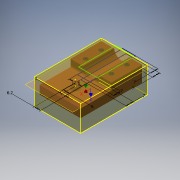
# Autodesk Inventor part: 17-0028-0109
Saved by Autodesk Inventor 2016 SP2 (Build 200236200, 236)
## iProperties
Created: 2017-12-29
Part Number: 17-0028-0109
Material: Copper
Document SubType Name: Modeling
Designer: Daan Giesen
Density: 8.94 g/cm^3
Appearance: Copper - Satin
Project: Digital PID Loop
Cost Center: 17-0028
User Status: CNC
Authority: Reichsöllner, Lukas
Mass: 216.263 g
Surface Area: 82.0629 cm^2
Volume: 24.1905 cm^3
Category: IOP
Company: Universiteit van Amsterdam
Author: Daan Giesen
Title: Digital PID Loop
Revision Number: A.1
Autodesk Inventor part; units mm, degrees
ref_plane "YZ Plane" through (0, 0, 0) normal (1, 0, 0) x (0, 1, 0)
ref_plane "XZ Plane" through (0, 0, 0) normal (0, 1, 0) x (-1, 0, 0)
sketch "Sketch1" plane through (0, 0, 0) normal (0, 0, 1) x (1, 0, 0)
  line L0 (0, 57) -> (0, -27) construction
  line L1 (-28, 0) -> (28, 0) construction
  line L2 (-20, 45) -> (20, 45)
  line L3 (20, 45) -> (20, -15)
  line L4 (20, -15) -> (-20, -15)
  line L5 (-20, -15) -> (-20, 45)
  line L6 (-20, 45) -> (20, -15) construction
  line L7 (20, 45) -> (-20, -15) construction
  point P0 (0, 0)
  point P1 (0, 15)
  dimension "d0" = 60
  dimension "d1" = 40
  dimension "d2" = 15
  constraints: 12 end point, 3 midpoint, 2 parallel, 1 horizontal, 1 perpendicular
  measures "d0" distance of L4.end L2.start
  measures "d1" distance of L3.end L4.end
  measures "d2" distance from line of L4 point (0, 0)
extrude "Extrusion1" add sketch "Sketch1" along normal blind 8
sketch "Sketch2" plane through (0, 0, 8) normal (0, 0, 1) x (1, 0, 0)
  point P0 (0, 0)
  point P1 (0, 0)
  constraints: 1 coincident
hole "Hole1" at (0, 0, 8) direction (0, 0, -1) diameter 8 end through all
sketch "Sketch3" plane through (0, 0, 8) normal (0, 0, 1) x (1, 0, 0)
  line L0 (-20, 15) -> (20, 15)
  line L1 (20, 15) -> (20, 45)
  line L2 (20, 45) -> (-20, 45)
  line L3 (-20, 45) -> (-20, 15)
  line L4 (-20, 15) -> (20, 45) construction
  line L5 (20, 15) -> (-20, 45) construction
  circle A0 centre (0, 0) radius 4 projected
  line L6 (20, 45) -> (-20, 45) projected
  line L7 (-20, 45) -> (-20, -15) projected
  line L8 (-20, -15) -> (20, -15) projected
  line L9 (20, -15) -> (20, 45) projected
  point P0 (0, 30)
  dimension "d12" = 30
  constraints: 12 end point, 2 midpoint, 2 parallel, 1 horizontal, 1 perpendicular
  measures "d12" distance between parallel lines of L2 L0
extrude "Extrusion2" add sketch "Sketch3" along normal blind 7 contours L3 L2 L1 L0
sketch "Sketch4" plane through (-20, 45, 0) normal (0, 1, 0) x (1, 0, 0)
  circle A0 centre (20, -16) radius 7.5
  line L0 (40, -15) -> (0, -15) projected
  line L1 (0, 0) -> (40, 0) projected
  point P0 (20, 0)
  point P1 (20, 0)
  dimension "d15" = 1
  dimension "d16" = 15
  constraints: 1 centre point, 1 midpoint, 1 vertical alignment
  measures "d15" distance from line of L0 A0.centre
  measures "d16" diameter of A0
extrude "Extrusion3" cut sketch "Sketch4" against normal through all
sketch "Sketch5" plane through (0, 0, 15) normal (0, 0, 1) x (1, 0, 0)
  point P0 (12.5, 22.5)
  point P1 (-12.5, 22.5)
  point P2 (-12.5, 37.5)
  point P3 (12.5, 37.5)
hole "Hole2" at (12.5, 22.5, 15) at (-12.5, 22.5, 15) at (-12.5, 37.5, 15) at (12.5, 37.5, 15) direction (0, 0, -1) diameter 4.134 depth 19.7 tip angle 120 thread size "M5x0.8" class "6H" standard "ISO Metric profile"
ref_plane "Work Plane1" through (0, 0, 12.2) normal (0, 0, 1) x (1, 0, 0)
sketch "Sketch6" plane through (0, 0, 12.2) normal (0, 0, 1) x (1, 0, 0)
  line L0 (6.2, 52) -> (-6.2, 52)
  line L1 (-6.2, 52) -> (-6.2, 8)
  line L2 (-6.2, 8) -> (6.2, 8)
  line L3 (6.2, 8) -> (6.2, 52)
  line L4 (20, 45) -> (7.433, 45) projected
  line L5 (7.433, 15) -> (20, 15) projected
  point P0 (0, 0)
  dimension "d27" = 12.4
  dimension "d28" = 6.2
  dimension "d29" = 7
  dimension "d30" = 7
  constraints: 8 end point, 2 parallel, 1 horizontal, 1 perpendicular
  measures "d27" distance of L2.end L1.end
  measures "d28" distance from line of L3 point (0, 0)
  measures "d29" distance between parallel lines of L4 L0
  measures "d30" distance between parallel lines of L5 L2
ref_plane "Work Plane2" through (0, 0, 9.5) normal (0, 0, 1) x (1, 0, 0)
sketch "Sketch7" plane through (0, 0, 9.5) normal (0, 0, 1) x (1, 0, 0)
  line L0 (3, 52) -> (-3, 52)
  line L1 (-3, 52) -> (-3, 8)
  line L2 (-3, 8) -> (3, 8)
  line L3 (3, 8) -> (3, 52)
  line L4 (7.433, 15) -> (20, 15) projected
  line L5 (20, 45) -> (7.433, 45) projected
  point P0 (0, 0)
  dimension "d32" = 6
  dimension "d33" = 7
  dimension "d35" = 7
  dimension "d36" = 3
  constraints: 8 end point, 2 parallel, 1 horizontal, 1 perpendicular
  measures "d32" distance of L1.end L2.end
  measures "d33" distance between parallel lines of L4 L2
  measures "d35" distance between parallel lines of L5 L0
  measures "d36" distance from line of point (0, 0) L3
sketch "Sketch8" plane through (0, 0, 15) normal (0, 0, 1) x (1, 0, 0)
  line L0 (8.9779, 48.2362) -> (-9.2966, 48.2362)
  line L1 (-9.2966, 48.2362) -> (-9.2966, 12.2184)
  line L2 (-9.2966, 12.2184) -> (8.9779, 12.2184)
  line L3 (8.9779, 12.2184) -> (8.9779, 48.2362)
  point P0 (0, 0)
  constraints: 8 end point, 2 parallel, 1 horizontal, 1 perpendicular
chamfer "Chamfer1" distance 0.25 angle 45 6 edges at (-20, 15, 11.5) (-20, 45, 7.5) (-20, -15, 4) (20, 45, 7.5) (20, 15, 11.5) (20, -15, 4)
body "Solid1"
